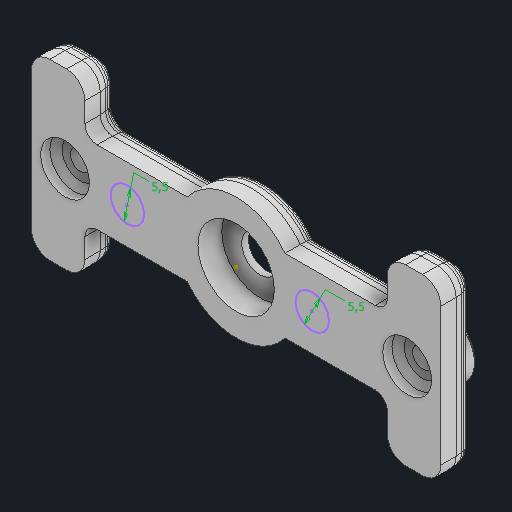
# Autodesk Inventor part: EndEffector_Holder
Saved by Autodesk Inventor 2025.2 (Build 292293000, 293)
## iProperties
Created: 2025-07-03
Part Number: EndEffector_Holder
Material: Generic
Document SubType Name: Modeling
Designer: Tiago
Density: 1 g/cm^3
Appearance: Default
Author: Tiago
Autodesk Inventor part; units mm, degrees
ref_plane "YZ Plane" through (0, 0, 0) normal (1, 0, 0) x (0, 1, 0)
ref_plane "XZ Plane" through (0, 0, 0) normal (0, 1, 0) x (-1, 0, 0)
ref_plane "XY Plane" through (0, 0, 0) normal (0, 0, 1) x (1, 0, 0)
sketch "Sketch1" plane through (0, 0, 0) normal (0, 0, 1) x (1, 0, 0)
  line L0 (33.5, -11.25) -> (33.5, 11.25)
  line L1 (-33.5, 11.25) -> (-33.5, -11.25)
  circle A0 centre (-29.25, 10) radius 1.75
  circle A1 centre (29.25, 10) radius 1.75
  circle A2 centre (-29.25, -10) radius 1.75
  circle A3 centre (29.25, -10) radius 1.75
  circle A4 centre (0, 0) radius 6.25
  arc A5 (-30.5, 14.25) -> (-33.5, 11.25) centre (-30.5, 11.25) ccw
  arc A6 (-33.5, -11.25) -> (-30.5, -14.25) centre (-30.5, -11.25) ccw
  arc A7 (30.5, -14.25) -> (33.5, -11.25) centre (30.5, -11.25) ccw
  arc A8 (33.5, 11.25) -> (30.5, 14.25) centre (30.5, 11.25) ccw
  line L2 (-24.75, 8) -> (-24.75, 11.25)
  line L3 (24.75, 8) -> (24.75, 11.25)
  line L4 (30.5, 14.25) -> (27.75, 14.25)
  line L5 (-27.75, 14.25) -> (-30.5, 14.25)
  line L6 (-30.5, -14.25) -> (-27.75, -14.25)
  line L7 (27.75, -14.25) -> (30.5, -14.25)
  arc A9 (27.75, 14.25) -> (24.75, 11.25) centre (27.75, 11.25) ccw
  arc A10 (24.75, -11.25) -> (27.75, -14.25) centre (27.75, -11.25) ccw
  arc A11 (-27.75, -14.25) -> (-24.75, -11.25) centre (-27.75, -11.25) ccw
  arc A12 (-24.75, 11.25) -> (-27.75, 14.25) centre (-27.75, 11.25) ccw
  circle A13 centre (0, 0) radius 3
  line L8 (0, 0) -> (0, 1.4867) construction
  line L9 (-22.75, 6) -> (22.75, 6)
  line L10 (-22.75, -6) -> (22.75, -6)
  arc A14 (22.75, 6) -> (24.75, 8) centre (22.75, 8) ccw
  arc A15 (-24.75, 8) -> (-22.75, 6) centre (-22.75, 8) ccw
  line L11 (-24.75, -11.25) -> (-24.75, -8)
  line L12 (24.75, -11.25) -> (24.75, -8)
  arc A16 (24.75, -8) -> (22.75, -6) centre (22.75, -8) ccw
  arc A17 (-22.75, -6) -> (-24.75, -8) centre (-22.75, -8) ccw
  circle A18 centre (28, 0) radius 2.5 construction
  circle A19 centre (28, 0) radius 5
  circle A20 centre (0, 0) radius 10
  point P0 (-33.5, 0)
  point P1 (33.5, 0)
  point P2 (-24.75, -6)
  point P3 (24.75, -6)
  point P4 (8, 6)
  point P5 (-8, 6)
  point P6 (-1.75, 6)
  point P7 (1.75, 6)
  point P8 (-8, -6)
  point P9 (8, -6)
  point P10 (1.75, -6)
  point P11 (-1.75, -6)
  point P12 (1.199, -2.75)
  point P13 (-1.199, -2.75)
  point P14 (-1.199, 2.75)
  point P15 (1.199, 2.75)
  dimension "d0" = 58.5
  dimension "d1" = 3.5
  dimension "d2" = 3.5
  dimension "d3" = 20
  dimension "FF" = 3.5
  dimension "d5" = 3.5
  dimension "d7" = 67
  dimension "d8" = 29.25
  dimension "d9" = 10
  dimension "d10" = 12.5
  dimension "d11" = 3
  dimension "d12" = 4.5
  dimension "d13" = 4.5
  dimension "d14" = 3
  dimension "d15" = 33.5
  dimension "d16" = 28.5
  dimension "d17" = 6
  dimension "d28" = 6
  dimension "d29" = 2
  dimension "d30" = 2
  dimension "d75" = 5
  dimension "d76" = 28
  dimension "d84" = 10
  dimension "d136" = 20
  dimension "d137" = 6
  constraints: 28 tangent, 26 end point, 24 point on circle, 21 centre point, 9 perpendicular, 8 equal radius, 8 point on line, 6 horizontal alignment, 5 parallel, 4 coincident, 2 horizontal, 2 midpoint, 2 vertical, 2 vertical alignment
  measures "d0" distance of A1.centre A0.centre
  measures "d1" diameter of A1
  measures "d2" diameter of A0
  measures "d3" distance of A0.centre A2.centre
  measures "FF" diameter of A2
  measures "d5" diameter of A3
  measures "d7" distance between parallel lines of L0 L1
  measures "d8" horizontal distance of point (0, 0) A1.centre
  measures "d9" vertical distance of point (0, 0) A1.centre
  measures "d10" diameter of A4
  measures "d11" radius of A5
  measures "d12" distance from line of A2.centre L2
  measures "d13" distance from line of A1.centre L3
  measures "d14" radius of A9
  measures "d15" distance from line of point (0, 0) L0
  measures "d16" distance between parallel lines of L7 L4
  measures "d17" diameter of A13
  measures "d28" distance from line of L9 point (0, 0)
  measures "d29" radius of A14
  measures "d30" radius of A16
  measures "d75" diameter of A18
  measures "d76" distance of A18.centre point (0, 0)
  measures "d84" diameter of A19
  measures "d136" diameter of A20
  measures "d137" distance from line of point (0, 0) L10
extrude "Extrusion1" add sketch "Sketch1" along normal blind 5 contours A7 L7 A10 L12 A16 L10 A20 L9 A14 L3 A9 L4 A8 L0 | L10 A4 L9 A20 | A20 L9 A4 L10 | L10 A17 L11 A11 L6 A6 L1 A5 L5 A12 L2 A15 L9 A20 | A19
extrude "Extrusion2" add sketch "Sketch1" along normal blind 5 contours A7 L7 A10 L12 A16 L10 A20 L9 A14 L3 A9 L4 A8 L0 | A20 L10 A4 | L10 A4 L9 A20 | L9 A4 A20 | L10 A4 L9 | A4 L10 | A20 L9 A4 L10 | L10 A17 L11 A11 L6 A6 L1 A5 L5 A12 L2 A15 L9 A20 | L9 A4 | A0 | A1 | A2 | A3 | A19
sketch "Sketch2" plane through (0, 0, 0) normal (0, 0, -1) x (-1, 0, 0)
  circle A0 centre (0, 0) radius 2.5
  circle A1 centre (0, 0) radius 10
  line L0 (22.75, -6) -> (-22.75, -6) projected
  line L1 (-8, -6) -> (8, -6)
  line L2 (-7.569, 13.3848) -> (-0.75, 13.3848)
  line L3 (0.75, 13.3848) -> (7.569, 13.3848)
  line L4 (-7.569, 13.3848) -> (-7.569, 6.5353)
  line L5 (7.569, 13.3848) -> (7.569, 6.5353)
  line L6 (0.75, 13.3848) -> (0.75, 2.3848)
  line L7 (-0.75, 13.3848) -> (-0.75, 2.9047)
  circle A2 centre (0, 0) radius 3 projected
  point P0 (0, 13.3848)
  point P1 (4.1595, 13.3848)
  point P2 (-4.1595, 13.3848)
  point P3 (-0.75, 9.9718)
  point P4 (0.75, 9.9718)
  point P5 (-0.75, 4.1071)
  point P6 (3.1414, -2.75)
  point P7 (-3.1414, -2.75)
  point P8 (0.75, 2.9047)
  point P9 (1.199, -2.75)
  point P10 (1.199, 2.75)
  dimension "d35" = 5
  dimension "d36" = 20
  dimension "d112" = 0.75
  dimension "d113" = 0.75
  dimension "d114" = 6.819
  dimension "d115" = 6.819
  dimension "d116" = 11
  constraints: 14 end point, 5 point on circle, 4 vertical, 3 coincident, 2 horizontal alignment, 2 midpoint, 1 centre point, 1 collinear, 1 horizontal, 1 vertical alignment, 6 other
  measures "d36" diameter of A1
  measures "d112" distance of L3.start point (0, 13.385)
  measures "d113" distance of point (0, 13.385) L2.end
  measures "d114" distance of L2.start L2.end
  measures "d115" distance of L3.start L3.end
  measures "d116" distance of L3.start L6.end
chamfer "Chamfer1" distance 1 angle 45 28 edges at (24.1642, 6.5858, 0) (15.375, 6, 0) (24.75, 9.625, 0) (25.6287, 13.3713, 0) (29.125, 14.25, 0) (32.6213, 13.3713, 0) (33.5, 0, 0) (32.6213, -13.3713, 0) (29.125, -14.25, 0) (25.6287, -13.3713, 0) (24.75, -9.625, 0) (24.1642, -6.5858, 0) (15.375, -6, 0) (-24.1642, 6.5858, 0) (-24.75, 9.625, 0) (-25.6287, 13.3713, 0) (-29.125, 14.25, 0) (-32.6213, 13.3713, 0) (-33.5, 0, 0) (-32.6213, -13.3713, 0) (-29.125, -14.25, 0) (-25.6287, -13.3713, 0) (-24.75, -9.625, 0) (-24.1642, -6.5858, 0) (-15.375, -6, 0) (-15.375, 6, 0) (0, 10, 0) (0, -10, 0)
sketch "Sketch6" plane through (0, 0, 5) normal (0, 0, 1) x (1, 0, 0)
  circle A0 centre (28, 0) radius 4
  circle A1 centre (28, 0) radius 1.65
  line L0 (0, -6.88) -> (0, 0) construction
  circle A2 centre (-28, 0) radius 4
  circle A3 centre (-28, 0) radius 1.65
  dimension "d77" = 28
  dimension "d78" = 8
  dimension "d81" = 3.3
  constraints: 4 centre point, 2 coincident, 2 end point, 2 symmetric about line, 1 horizontal alignment, 1 vertical, 2 other
  measures "d77" distance of L0.end A0.centre
  measures "d78" diameter of A0
  measures "d81" diameter of A1
extrude "Extrusion10" add sketch "Sketch1" along normal blind 1 and the other way blind 1.5 contours A19
mirror "Mirror2" about plane through (0, 0, 0) normal (1, 0, 0) of "Extrusion10"
chamfer "Chamfer5" distance 0.5 angle 45 2 edges at (-23, 0, -1.5) (23, 0, -1.5)
extrude "Extrusion11" cut sketch "Sketch6" against normal up to surface (6.5 mm away) contours A1 | A3
extrude "Extrusion12" cut sketch "Sketch6" against normal blind 2.5
fillet "Fillet3" radius 1 2 edges at (-23, 0, 0) (23, 0, 0)
chamfer "Chamfer7" distance 1 angle 45 2 edges at (-32, 0, 2.5) (24, 0, 2.5)
chamfer "Chamfer9" distance 0.5 angle 45 28 edges at (-24.1642, 6.5858, 1) (-15.375, 6, 1) (-24.75, 9.625, 1) (-25.6287, 13.3713, 1) (-29.125, 14.25, 1) (-32.6213, 13.3713, 1) (-33.5, 0, 1) (-32.6213, -13.3713, 1) (-29.125, -14.25, 1) (-25.6287, -13.3713, 1) (-24.75, -9.625, 1) (-24.1642, -6.5858, 1) (-15.375, -6, 1) (24.1642, 6.5858, 1) (24.75, 9.625, 1) (25.6287, 13.3713, 1) (29.125, 14.25, 1) (32.6213, 13.3713, 1) (33.5, 0, 1) (32.6213, -13.3713, 1) (29.125, -14.25, 1) (25.6287, -13.3713, 1) (24.75, -9.625, 1) (24.1642, -6.5858, 1) (15.375, -6, 1) (15.375, 6, 1) (0, 10, 1) (0, -10, 1)
chamfer "Chamfer10" distance 0.5 angle 45 28 edges at (-24.1642, 6.5858, 1.5) (-15.375, 6, 1.5) (-24.75, 9.625, 1.5) (-25.6287, 13.3713, 1.5) (-29.125, 14.25, 1.5) (-32.6213, 13.3713, 1.5) (-33.5, 0, 1.5) (-32.6213, -13.3713, 1.5) (-29.125, -14.25, 1.5) (-25.6287, -13.3713, 1.5) (-24.75, -9.625, 1.5) (-24.1642, -6.5858, 1.5) (-15.375, -6, 1.5) (24.1642, 6.5858, 1.5) (24.75, 9.625, 1.5) (25.6287, 13.3713, 1.5) (29.125, 14.25, 1.5) (32.6213, 13.3713, 1.5) (33.5, 0, 1.5) (32.6213, -13.3713, 1.5) (29.125, -14.25, 1.5) (25.6287, -13.3713, 1.5) (24.75, -9.625, 1.5) (24.1642, -6.5858, 1.5) (15.375, -6, 1.5) (15.375, 6, 1.5) (0, -10, 1.5) (0, 10, 1.5)
chamfer "Chamfer11" distance 0.5 angle 45 28 edges at (-24.1642, 6.5858, 2) (-15.375, 6, 2) (-24.75, 9.625, 2) (-25.6287, 13.3713, 2) (-29.125, 14.25, 2) (-32.6213, 13.3713, 2) (-33.5, 0, 2) (-32.6213, -13.3713, 2) (-29.125, -14.25, 2) (-25.6287, -13.3713, 2) (-24.75, -9.625, 2) (-24.1642, -6.5858, 2) (-15.375, -6, 2) (24.1642, 6.5858, 2) (24.75, 9.625, 2) (25.6287, 13.3713, 2) (29.125, 14.25, 2) (32.6213, 13.3713, 2) (33.5, 0, 2) (32.6213, -13.3713, 2) (29.125, -14.25, 2) (25.6287, -13.3713, 2) (24.75, -9.625, 2) (24.1642, -6.5858, 2) (15.375, -6, 2) (15.375, 6, 2) (0, -10, 2) (0, 10, 2)
sketch "Sketch8" plane through (0, 0, 5) normal (0, 0, 1) x (1, 0, 0)
  circle A0 centre (0, 0) radius 6.25
  dimension "d138" = 12.5
  constraints: 1 centre point, 1 coincident
  measures "d138" diameter of A0
extrude "Extrusion15" cut sketch "Sketch8" against normal blind 3.9
sketch "Sketch10" plane through (0, 0, 5) normal (0, 0, 1) x (1, 0, 0)
  circle A0 centre (12.4533, 0) radius 2.75
  circle A1 centre (-17.799, 0) radius 2.75
  point P0 (0, 0)
  dimension "d145" = 5.5
  dimension "d146" = 5.5
  constraints: 2 centre point
  measures "d145" diameter of A1
  measures "d146" diameter of A0
equation "\"d1\" = FF"
equation "\"d2\" = FF"
equation "\"d5\" = FF"
body "Solid1"
